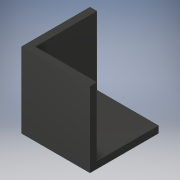
# Autodesk Inventor part: batteryCornerMount
Saved by Autodesk Inventor 2017 (Build 210142000, 142)
## iProperties
Created: 2020-02-01
Part Number: batteryCornerMount
Material: UHMW, Black
Document SubType Name: Modeling
Designer: S338674153
Density: 0.94 g/cm^3
Appearance: Smooth - Black
Author: S338674153
Autodesk Inventor part; units mm, degrees
ref_plane "YZ Plane" through (0, 0, 0) normal (1, 0, 0) x (0, 1, 0)
ref_plane "XZ Plane" through (0, 0, 0) normal (0, 1, 0) x (-1, 0, 0)
ref_plane "XY Plane" through (0, 0, 0) normal (0, 0, 1) x (1, 0, 0)
sketch "Sketch1" plane through (0, 0, 0) normal (0, 1, 0) x (-1, 0, 0)
  line L0 (0, 0) -> (25.4, 0)
  line L1 (25.4, 0) -> (25.4, -25.4)
  line L2 (25.4, -25.4) -> (0, -25.4)
  line L3 (0, -25.4) -> (0, 0)
  dimension "d0" = 25.4
  dimension "d1" = 25.4
  constraints: 8 end point, 2 parallel, 1 horizontal, 1 perpendicular
  measures "d0" distance of L1.end L2.end
  measures "d1" distance of L0.end L1.end
extrude "Extrusion1" add sketch "Sketch1" along normal blind 2.54
sketch "Sketch2" plane through (0, 2.54, 0) normal (0, 1, 0) x (1, 0, 0)
  line L0 (-25.4, 0) -> (0, 0) projected
  line L1 (-25.4, 25.4) -> (-25.4, 0) projected
  line L2 (0, 0) -> (-25.4, 0)
  line L3 (-25.4, 0) -> (-25.4, 2.5321)
  line L4 (-22.86, 2.5321) -> (0, 2.5321)
  line L5 (0, 2.5321) -> (0, 0)
  line L6 (0, 25.4) -> (-25.4, 25.4) projected
  line L7 (-25.4, 0) -> (-22.86, 0)
  line L8 (-22.86, 2.5321) -> (-22.86, 25.4)
  line L9 (-22.86, 25.4) -> (-25.4, 25.4)
  line L10 (-25.4, 25.4) -> (-25.4, 0)
  dimension "d4" = 2.54
  constraints: 16 end point, 4 parallel, 2 horizontal, 2 perpendicular, 2 point on line
  measures "d4" distance of L9.end L8.end
extrude "Extrusion2" add sketch "Sketch2" along normal blind 25.4
body "Solid1"
